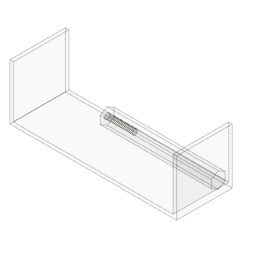
Ascender v2 (Autodesk Fusion 360 design; units mm, degrees)
Autodesk Fusion 360 part; units mm, degrees
sketch "Sketch1" plane through (0, 0, 0) normal (0, 1, 0) x (1, 0, 0) in component "Winch Baseplate"
  line L0 (88.9, -60.96) -> (88.9, -10.16)
  line L1 (88.9, -10.16) -> (-63.5, -10.16)
  line L2 (-63.5, -10.16) -> (-63.5, -60.96)
  line L3 (85.725, -57.785) -> (85.725, -13.335)
  line L4 (85.725, -13.335) -> (-60.325, -13.335)
  line L5 (-60.325, -13.335) -> (-60.325, -57.785)
  line L6 (-60.325, -57.785) -> (-60.325, -60.96)
  line L7 (85.725, -57.785) -> (85.725, -60.96)
  line L8 (-63.5, -60.96) -> (-60.325, -60.96)
  line L9 (85.725, -60.96) -> (88.9, -60.96)
  dimension "d1" = 152.4
  dimension "d2" = 50.8
  constraint horizontal L8
  constraint vertical L0
  constraint horizontal L1
  constraint vertical L2
  constraint perpendicular L6 L8
  constraint coincident L7.end L8
  constraint perpendicular L7 L8
  constraint collinear L8 L9
  measures "d1" distance of L2.end L0.start
  measures "d2" distance of L2.end L1.end
extrude "Extrude1" add sketch "Sketch1" along normal blind 50.8 makes body 1 in component "Winch Baseplate"
sketch "Sketch1 (2)" plane through (0, 0, 0) normal (1, 0, 0) x (0, 1, 0) in component "Winch Axle Extension"
  line L0 (50.8, 60.96, -63.5) -> (0, 10.16, -63.5)
  line L1 (50.8, 10.16) -> (0, 60.96)
  line L2 (19.05, 31.8938) -> (25.4, 28.2277)
  line L3 (25.4, 28.2277) -> (31.75, 31.8938)
  line L4 (31.75, 31.8938) -> (31.75, 39.2262)
  line L5 (31.75, 39.2262) -> (25.4, 42.8923)
  line L6 (25.4, 42.8923) -> (19.05, 39.2262)
  line L7 (19.05, 39.2262) -> (19.05, 31.8938)
  point P0 (25.4, 35.56)
  dimension "d7" = 6.35
  constraint midpoint L1 P0
  measures "d7" distance of P0 L7
extrude "Extrude1'" add sketch "Sketch1 (2)" along normal blind 101.6 separate body makes body 2 in component "Winch Axle Extension"
sketch "Sketch2" plane through (0, 0, 0) normal (-1, 0, 0) x (0, -1, 0) in component "Winch Axle Extension"
  line L0 (-19.05, 31.8938) -> (-19.05, 39.2262)
  line L1 (-19.05, 39.2262) -> (-25.4, 42.8923)
  line L2 (-25.4, 42.8923) -> (-31.75, 39.2262)
  line L3 (-31.75, 39.2262) -> (-31.75, 31.8938)
  line L4 (-31.75, 31.8938) -> (-25.4, 28.2277)
  line L5 (-25.4, 28.2277) -> (-19.05, 31.8938)
  line L6 (-31.75, 39.2262) -> (-19.05, 31.8938)
  circle A0 centre (-25.4, 35.56) radius 3.175
  dimension "d10" = 6.35
  constraint coincident L2.end L3.start
  constraint coincident L0.start L5.end
  constraint midpoint L6 A0.centre
  measures "d10" diameter of A0
hole "Hole1" at (0, 25.4, 35.56) direction (1, 0, 0) diameter 5.1308 depth 25.4 tip angle 180 bodies 2 in component "Winch Axle Extension"
thread "Thread1" "ANSI Unified Screw Threads 0.25 1/4-20 UNC 1B" in component "Winch Axle Extension"
sketch "Sketch1 (3)" plane through (0, 0, 0) normal (1, 0, 0) x (0, 1, 0) in component "Winch Axle Connection"
component "Winch" placed x (1, 0, 0) y (0, 1, 0) z (0, 0, 1) at (0, 0, 0)
component "Winch Baseplate" placed x (1, 0, 0) y (0, 1, 0) z (0, 0, 1) at (0, 0, 0) in component "Winch"
component "Winch Axle Extension" placed x (1, 0, 0) y (0, 1, 0) z (0, 0, 1) at (0, 0, 0) in component "Winch"
component "Winch Axle Connection" placed x (1, 0, 0) y (0, 1, 0) z (0, 0, 1) at (0, 0, 0) in component "Winch Axle Extension"
